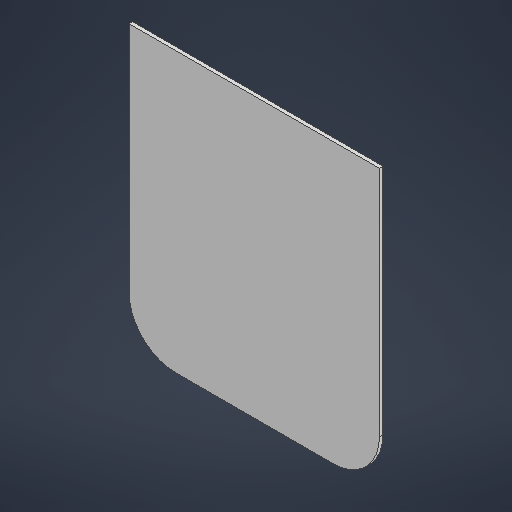
# Autodesk Inventor part: 屏幕
Saved by Autodesk Inventor 2025 (Build 290162000, 162)
## iProperties
Created: 2025-11-17
Part Number: 屏幕
Material: 常规
Document SubType Name: Modeling
Designer: XH
Density: 1 g/cm^3
Appearance: 默认
Author: XH
Autodesk Inventor part; units mm, degrees
ref_plane "YZ Plane" through (0, 0, 0) normal (1, 0, 0) x (0, 1, 0)
ref_plane "XZ Plane" through (0, 0, 0) normal (0, 1, 0) x (-1, 0, 0)
ref_plane "XY Plane" through (0, 0, 0) normal (0, 0, 1) x (1, 0, 0)
sketch "草图1" plane through (0, 0, 0) normal (0, 0, 1) x (1, 0, 0)
  line L0 (35, -39) -> (-35, -39)
  line L1 (-35, -39) -> (-35, 39)
  line L2 (-35, 39) -> (35, 39)
  line L3 (35, 39) -> (35, -39)
  line L4 (35, -39) -> (-35, 39) construction
  line L5 (-35, -39) -> (35, 39) construction
  point P0 (0, 0)
  dimension "d0" = 70
  dimension "d1" = 78
  constraints: 12 end point, 2 midpoint, 2 parallel, 1 horizontal, 1 perpendicular
  measures "d0" distance of L1.end L2.end
  measures "d1" distance of L2.end L0.start
extrude "拉伸1" add sketch "草图1" along normal blind 1
fillet "圆角1" radius 13 2 edges at (-35, -39, 0.5) (35, -39, 0.5)
